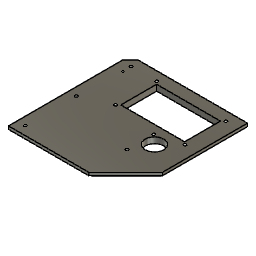
ECE198 Housing v1-11 (Autodesk Fusion 360 archive; units mm, degrees)
design "Lid"
Autodesk Fusion 360 part; units mm, degrees
other "DerivedContext1"
sketch "lid v2" plane through (-180, 0, 0) normal (0, 0, 1) x (1, 0, 0)
  line L0 (334.0338, -3.2613) -> (192.2917, -3.2613)
  line L1 (316.9875, -15.8281) -> (316.9875, -64.0063)
  line L2 (287.0338, -159.4636) -> (334.0338, -112.4636)
  line L3 (231.1593, -15.8281) -> (316.9875, -15.8281)
  line L4 (337.6529, -114.5635) -> (288.1529, -164.0635)
  line L5 (192.2917, -3.2613) -> (183.2917, -12.2613)
  line L6 (334.0338, -112.4636) -> (334.0338, -3.2613)
  line L7 (183.2917, -12.2613) -> (183.2917, -159.4636)
  line L8 (316.9875, -64.0063) -> (231.1593, -64.0063)
  line L9 (183.2917, -159.4636) -> (287.0338, -159.4636)
  line L10 (180, -164.0635) -> (180, -10.5)
  line L11 (288.1529, -164.0635) -> (180, -164.0635)
  line L12 (180, -10.5) -> (190.5, 0)
  line L13 (337.6529, 0) -> (337.6529, -114.5635)
  line L14 (190.5, 0) -> (337.6529, 0)
  circle A0 centre (299.8198, -87.3938) radius 12.5
  line L15 (231.1593, -64.0063) -> (231.1593, -15.8281)
extrude "Extrude3" add sketch "lid v2" along normal blind 4 contours L0 L2 L5 L6 L7 L9 | L4 L10 L11 L12 L13 L14
sketch "holes" plane through (0, 0, 0) normal (0, 0, 1) x (1, 0, 0)
  circle A0 through (105.4825, -111.8847, 4) (108.2372, -113.4751, 4) (108.2372, -110.2943, 4)
  circle A1 through (45.6664, -67.3964, 4) (48.4211, -68.9868, 4) (48.4211, -65.8059, 4)
  circle A2 through (31.3204, -70.8602, 4) (32.826, -71.7295, 4) (32.826, -69.991, 4)
  circle A3 through (138.8906, -67.3151, 4) (141.6453, -68.9056, 4) (141.6453, -65.7247, 4)
  circle A4 through (31.3204, -31.7681, 4) (32.826, -32.6373, 4) (32.826, -30.8988, 4)
  circle A5 through (8.9685, -83.5722, 4) (11.7232, -85.1627, 4) (11.7232, -81.9818, 4)
  circle A6 through (31.3204, -70.8602, 4) (32.826, -71.7295, 4) (32.826, -69.991, 4)
  circle A7 through (45.6664, -67.3964, 4) (48.4211, -68.9868, 4) (48.4211, -65.8059, 4)
  circle A8 through (12.1917, -23.4202, 4) (14.3474, -24.6648, 4) (14.3474, -22.1757, 4)
  circle A9 through (9.0147, -152.3487, 4) (11.7694, -153.9392, 4) (11.7694, -150.7583, 4)
  circle A10 through (138.889, -12.2643, 4) (141.6437, -13.8547, 4) (141.6437, -10.6739, 4)
  circle A11 through (45.7204, -12.2533, 4) (48.4751, -13.8438, 4) (48.4751, -10.6629, 4)
  circle A12 through (10.9466, -31.7681, 4) (12.4522, -32.6373, 4) (12.4522, -30.8988, 4)
  circle A13 through (45.6664, -67.3964, 4) (48.4211, -68.9868, 4) (48.4211, -65.8059, 4)
  circle A14 through (11.4414, -12.3099, 4) (14.1961, -13.9003, 4) (14.1961, -10.7194, 4)
  circle A15 through (105.5452, -76.1037, 4) (108.2999, -77.6942, 4) (108.2999, -74.5133, 4)
  circle A16 through (10.9466, -70.8602, 4) (12.4522, -71.7295, 4) (12.4522, -69.991, 4)
  circle A17 through (45.6664, -67.3964, 4) (48.4211, -68.9868, 4) (48.4211, -65.8059, 4)
extrude "Extrude4" add sketch "lid v2" against normal blind 4 contours L0 L2 L5 L6 L7 L9
move_face "OffsetFaces1" offset -1 6 faces at (37.8724, -159.4636, -1.3333) (3.2917, -61.3287, -2.6667) (106.7864, -3.2613, -1.3333) (9.2917, -6.2613, -1.3333) (154.0338, -76.0628, -2.6667) (122.7004, -143.7969, -2.6667)
hole "Hole1" at (13.2779, -12.3099, 4) at (47.5029, -67.3964, 4) at (10.8512, -152.3487, 4) at (107.319, -111.8847, 4) at (107.3816, -76.1037, 4) at (140.7271, -67.3151, 4) at (140.7255, -12.2643, 4) at (10.805, -83.5722, 4) at (47.5569, -12.2533, 4) direction (0, 0, -1) diameter 3.783 depth 15 tip angle 180
thread "Thread1" "ISO Metric profile 4.5 M4.5x0.75 6H" major diameter 4.6131 minor diameter 3.7831 pitch 0.75 angle 60 resizes the face on face at (139.9924, -69.0581, 1.3333) on face at (13.4662, -14.192, -1.3333) on face at (9.2161, -84.5985, 1.3333) on face at (108.9079, -110.8585, 1.3333) on face at (108.9705, -75.0775, 1.3333) on face at (47.6512, -10.3642, 1.3333) on face at (45.914, -68.4226, 1.3333) on face at (8.9744, -152.5839, 1.3333) on face at (139.5097, -13.7133, 1.3333)
hole "Hole2" at (13.6288, -23.4202, 4) direction (0, 0, -1) diameter 3 depth 8 tip angle 180
